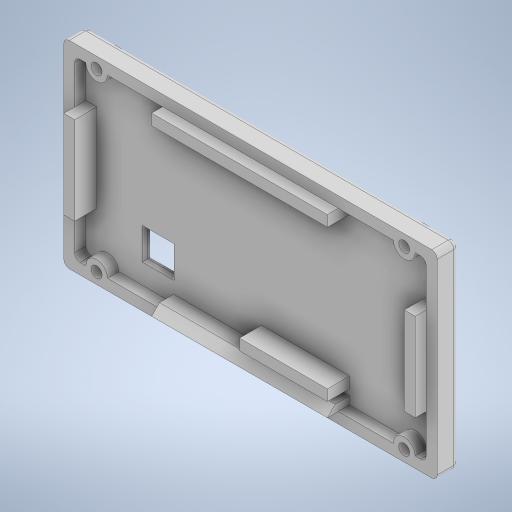
# Autodesk Inventor part: Case_Rear
Saved by Autodesk Inventor 2023 (Build 270158000, 158)
## iProperties
Created: 2022-12-07
Part Number: Case_Rear
Material: Generic
Document SubType Name: Modeling
Designer: elect
Density: 1 g/cm^3
Appearance: Default
Author: elect
Autodesk Inventor part; units mm, degrees
ref_plane "YZ Plane" through (0, 0, 0) normal (1, 0, 0) x (0, 1, 0)
ref_plane "XZ Plane" through (0, 0, 0) normal (0, 1, 0) x (-1, 0, 0)
ref_plane "XY Plane" through (0, 0, 0) normal (0, 0, 1) x (1, 0, 0)
sketch "Sketch1" plane through (0, 0, 0) normal (0, 0, 1) x (1, 0, 0)
  line L0 (1.5875, 0) -> (106.3625, 0)
  line L1 (107.95, 1.5875) -> (107.95, 55.5625)
  line L2 (106.3625, 57.15) -> (1.5875, 57.15)
  line L3 (0, 55.5625) -> (0, 1.5875)
  arc A0 (1.5875, 57.15) -> (0, 55.5625) centre (1.5875, 55.5625) ccw
  arc A1 (107.95, 55.5625) -> (106.3625, 57.15) centre (106.3625, 55.5625) ccw
  arc A2 (106.3625, 0) -> (107.95, 1.5875) centre (106.3625, 1.5875) ccw
  arc A3 (0, 1.5875) -> (1.5875, 0) centre (1.5875, 1.5875) ccw
  point P0 (0, 0)
  point P1 (107.95, 0)
  point P2 (0, 57.15)
  dimension "d0" = 57.15
  dimension "d1" = 107.95
  dimension "d2" = 1.5875
  dimension "d3" = 1.5875
  constraints: 8 end point, 8 point on circle, 8 tangent, 6 point on line, 4 centre point, 2 equal radius, 2 parallel, 1 horizontal, 1 perpendicular
  measures "d0" distance of point (0, 57.15) point (0, 0)
  measures "d1" distance of point (0, 0) point (107.95, 0)
  measures "d2" radius of A0
  measures "d3" radius of A1
extrude "Extrusion1" add sketch "Sketch1" along normal blind 6.35
sketch "Sketch2" plane through (0, 0, 6.35) normal (0, 0, 1) x (1, 0, 0)
  line L0 (104.775, 52.3875) -> (104.775, 4.7625)
  line L1 (3.175, 4.7625) -> (3.175, 52.3875)
  arc A0 (4.7625, 53.975) -> (3.175, 52.3875) centre (4.7625, 52.3875) ccw
  arc A1 (104.775, 52.3875) -> (103.1875, 53.975) centre (103.1875, 52.3875) ccw
  arc A2 (103.1875, 3.175) -> (104.775, 4.7625) centre (103.1875, 4.7625) ccw
  arc A3 (3.175, 4.7625) -> (4.7625, 3.175) centre (4.7625, 4.7625) ccw
  line L2 (106.3625, 57.15) -> (1.5875, 57.15) projected
  line L3 (107.95, 1.5875) -> (107.95, 55.5625) projected
  line L4 (1.5875, 0) -> (106.3625, 0) projected
  line L5 (0, 55.5625) -> (0, 1.5875) projected
  arc A4 (6.35, 53.975) -> (12.7, 53.975) centre (9.525, 53.975) ccw
  arc A5 (95.25, 53.975) -> (101.6, 53.975) centre (98.425, 53.975) ccw
  arc A6 (101.6, 3.175) -> (95.25, 3.175) centre (98.425, 3.175) ccw
  arc A7 (12.7, 3.175) -> (6.35, 3.175) centre (9.525, 3.175) ccw
  line L6 (4.7625, 53.975) -> (6.35, 53.975)
  line L7 (12.7, 53.975) -> (95.25, 53.975)
  line L8 (101.6, 53.975) -> (103.1875, 53.975)
  line L9 (103.1875, 3.175) -> (101.6, 3.175)
  line L10 (95.25, 3.175) -> (12.7, 3.175)
  line L11 (6.35, 3.175) -> (4.7625, 3.175)
  point P0 (0, 0)
  dimension "d6" = 1.5875
  dimension "d8" = 3.175
  dimension "d10" = 3.175
  dimension "d11" = 6.35
  dimension "d12" = 6.35
  dimension "d43" = 3.175
  constraints: 16 end point, 16 point on circle, 16 tangent, 10 parallel, 8 centre point, 6 equal radius, 3 horizontal, 3 perpendicular, 2 vertical alignment
  measures "d6" radius of A0
  measures "d8" distance between parallel lines of L3 L0
  measures "d10" distance between parallel lines of L5 L1
  measures "d11" distance from line of L1 A4.centre
  measures "d12" distance from line of L0 A5.centre
  measures "d43" radius of A4
extrude "Extrusion2" cut sketch "Sketch2" against normal blind 3.175
fillet "Fillet1" radius 1.5875 8 edges at (0.465, 56.685, 0) (0, 28.575, 0) (0.465, 0.465, 0) (53.975, 0, 0) (107.485, 0.465, 0) (107.95, 28.575, 0) (107.485, 56.685, 0) (53.975, 57.15, 0)
sketch "Sketch3" plane through (0, 0, 3.175) normal (0, 0, 1) x (1, 0, 0)
  line L0 (28.575, 54.0321) -> (79.375, 54.0321)
  line L1 (79.375, 54.0321) -> (79.375, 50.8571)
  line L2 (79.375, 50.8571) -> (28.575, 50.8571)
  line L3 (28.575, 50.8571) -> (28.575, 54.0321)
  line L4 (3.175, 4.7625) -> (3.175, 52.3875) projected
  line L5 (3.175, 41.275) -> (6.35, 41.275)
  line L6 (6.35, 41.275) -> (6.35, 15.875)
  line L7 (6.35, 15.875) -> (3.175, 15.875)
  line L8 (3.175, 15.875) -> (3.175, 41.275)
  line L9 (104.775, 52.3875) -> (104.775, 4.7625) projected
  line L10 (104.775, 41.275) -> (101.6, 41.275)
  line L11 (101.6, 41.275) -> (101.6, 15.875)
  line L12 (101.6, 15.875) -> (104.775, 15.875)
  line L13 (104.775, 15.875) -> (104.775, 41.275)
  line L14 (95.25, 3.175) -> (12.7, 3.175) projected
  line L15 (79.375, 3.175) -> (28.575, 3.175)
  line L16 (28.575, 3.175) -> (28.575, 5.461)
  line L17 (28.575, 5.461) -> (79.375, 5.461)
  line L18 (79.375, 5.461) -> (79.375, 3.175)
  line L19 (103.1875, 3.175) -> (101.6, 3.175) projected
  line L20 (101.6, 53.975) -> (103.1875, 53.975) projected
  point P0 (0, 0)
  point P1 (28.575, 4.318)
  point P2 (79.375, 4.318)
  point P3 (79.375, 52.4446)
  point P4 (4.7625, 41.275)
  point P5 (103.1875, 41.275)
  point P6 (103.1875, 15.875)
  point P7 (4.7625, 15.875)
  point P8 (102.3937, 3.175)
  dimension "d16" = 25.4
  dimension "d17" = 25.4
  dimension "d18" = 2.286
  dimension "d19" = 3.175
  dimension "d20" = 3.175
  dimension "d21" = 3.175
  dimension "d22" = 12.7
  dimension "d23" = 12.7
  constraints: 32 end point, 8 midpoint, 8 parallel, 4 horizontal, 4 perpendicular, 3 point on line, 2 horizontal alignment, 2 vertical alignment
  measures "d16" distance between parallel lines of L4 L16
  measures "d17" distance between parallel lines of L9 L18
  measures "d18" distance of L17.end L15.start
  measures "d19" distance between parallel lines of L2 L0
  measures "d20" distance of L5.start L5.end
  measures "d21" distance of L10.start L10.end
  measures "d22" distance from line of point (102.394, 3.175) L12
  measures "d23" distance between parallel lines of L20 L10
extrude "Extrusion3" add sketch "Sketch3" along normal blind 6.35
hole "Hole1" at (9.525, 53.975, 6.35) at (98.425, 53.975, 6.35) at (98.425, 3.175, 6.35) at (9.525, 3.175, 6.35) direction (0, 0, -1) diameter 3.175 end through all
sketch "Sketch5" plane through (0, 0, 0) normal (0, 0, -1) x (-1, 0, 0)
  line L0 (-28.702, 18.2245) -> (-19.558, 18.2245)
  line L1 (-19.558, 18.2245) -> (-19.558, 9.0805)
  line L2 (-19.558, 9.0805) -> (-28.702, 9.0805)
  line L3 (-28.702, 9.0805) -> (-28.702, 18.2245)
  line L4 (-1.5875, 1.5875) -> (-106.3625, 1.5875) projected
  line L5 (-1.5875, 55.5625) -> (-1.5875, 1.5875) projected
  point P0 (0, 0)
  point P1 (-24.13, 9.0805)
  dimension "d36" = 7.493
  dimension "d37" = 17.9705
  dimension "d38" = 9.144
  dimension "d39" = 9.144
  constraints: 8 end point, 2 parallel, 1 horizontal, 1 midpoint, 1 perpendicular
  measures "d36" distance from line of L4 point (-24.13, 9.081)
  measures "d37" distance between parallel lines of L5 L1
  measures "d38" distance of L0.start L0.end
  measures "d39" distance of L2.end L0.start
extrude "Extrusion4" cut sketch "Sketch5" against normal blind 6.35
fillet "Fillet2" radius 1.5875 4 edges at (24.13, 18.2245, 0) (19.558, 13.6525, 0) (28.702, 13.6525, 0) (24.13, 9.0805, 0)
sketch "Sketch7" plane through (0, 0, 3.175) normal (0, 0, 1) x (1, 0, 0)
  line L0 (79.375, 7.239) -> (53.975, 7.239)
  line L1 (53.975, 7.239) -> (53.975, 10.414)
  line L2 (53.975, 10.414) -> (79.375, 10.414)
  line L3 (79.375, 10.414) -> (79.375, 7.239)
  line L4 (79.375, 3.175) -> (79.375, 6.35) projected
  line L5 (28.575, 5.461) -> (79.375, 5.461) projected
  point P0 (0, 0)
  point P1 (79.375, 5.461)
  dimension "d48" = 3.175
  dimension "d49" = 25.4
  dimension "d50" = 0
  dimension "d51" = 1.778
  constraints: 8 end point, 2 parallel, 1 horizontal, 1 perpendicular, 1 other
  measures "d48" distance of L2.end L0.start
  measures "d49" distance of L1.end L2.end
  measures "d50" distance between parallel lines of L4 L3
extrude "Extrusion6" add sketch "Sketch7" along normal blind 6.35
chamfer "Chamfer2" distance 2.286 angle 45 1 edges at (53.975, 5.461, 9.525)
sketch "Sketch8" plane through (0, 0, 0) normal (0, 0, -1) x (-1, 0, 0)
  circle A0 centre (-98.425, 53.975) radius 1.5875 projected
  circle A1 centre (-9.525, 53.975) radius 1.5875 projected
  circle A2 centre (-9.525, 3.175) radius 1.5875 projected
  arc A3 (-95.25, 3.175) -> (-101.6, 3.175) centre (-98.425, 3.175) ccw projected
  point P0 (0, 0)
  point P1 (-9.525, 1.5875)
  constraints: 4 coincident, 1 vertical alignment
hole "Hole2" at (98.425, 53.975, 0) at (9.525, 53.975, 0) at (9.525, 3.175, 0) at (98.425, 3.175, 0) direction (0, 0, 1) diameter 3.175 depth 6.35 tip angle 118 counterbore diameter 5.334 counterbore depth 2.54
body "Solid1"
